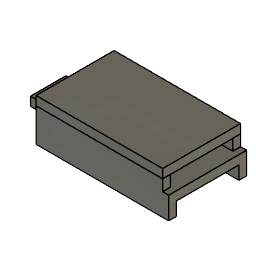
display (Autodesk Fusion 360 design; units mm, degrees)
Autodesk Fusion 360 part; units mm, degrees
note: some values were not read from the file. Chosen so that the rebuilt part matches the saved one: which bodies a step acts on; which face or edge a step refers to. Set by a fixed rule: which sketch regions a step uses.
sketch "スケッチ4" plane through (0, 0, 0) normal (0, 0, 1) x (1, 0, 0)
  line L0 (3, 8.75) -> (3, -8.75)
  line L1 (32.75, -8.75) -> (32.75, 8.75)
  line L2 (5, -8.75) -> (5, 8.75)
  line L3 (3, 8.75) -> (3, -8.75)
  line L4 (-3, -4) -> (-3, 4)
  circle A0 centre (0, 0) radius 1.75
  line L5 (32.75, 8.75) -> (32.75, -8.75)
  line L6 (30.75, 8.75) -> (32.75, 8.75)
  line L7 (32.75, 8.75) -> (3, 8.75)
  line L8 (3, -8.75) -> (32.75, -8.75)
  line L9 (32.75, -8.75) -> (30.75, -8.75)
  line L10 (30.75, -8.75) -> (30.75, 8.75)
  line L11 (-3, 4) -> (3, 4)
  line L12 (3, 4) -> (3, -4)
  line L13 (3, -8.75) -> (5, -8.75)
  line L14 (3, -4) -> (-3, -4)
  line L15 (5, 8.75) -> (3, 8.75)
  line L16 (32.75, 8.75) -> (32.75, -6.75)
  line L17 (3, 8.75) -> (34.75, 8.75)
  line L18 (34.75, 8.75) -> (34.75, 7)
  line L19 (34.75, 7) -> (3, 7)
  line L20 (3, 7) -> (3, 8.75)
  line L21 (30.75, 5) -> (32.75, 5)
  line L22 (32.75, 5) -> (32.75, -7)
  line L23 (32.75, -7) -> (30.75, -7)
  line L24 (30.75, -7) -> (30.75, 5)
  line L25 (3, -8.75) -> (32.75, -8.75)
  line L26 (32.75, -8.75) -> (32.75, -7)
  line L27 (32.75, -7) -> (3, -7)
  line L28 (3, -7) -> (3, -8.75)
  line L29 (34.75, 8.75) -> (31.4, 8.75)
  line L30 (31.4, 8.75) -> (31.4, -8.75)
  line L31 (31.4, -8.75) -> (34.75, -8.75)
  line L32 (34.75, -8.75) -> (34.75, 8.75)
  dimension "d19" = 3.5
  dimension "d20" = 6
  dimension "d21" = 8
  dimension "d22" = 4
  dimension "d23" = 3
  dimension "d24" = 17.5
  dimension "d25" = 8.75
  dimension "d26" = 29.75
  dimension "d33" = 2
  dimension "d34" = 2
  dimension "d35" = 1.75
  dimension "d38" = 2
  dimension "d39" = 1.75
  dimension "d40" = 3.35
  dimension "d41" = 17.5
  constraint coincident A0.centre origin
  constraint horizontal L11
  constraint vertical L12
  constraint horizontal L14
  constraint vertical L4
  constraint horizontal L8
  constraint vertical L1
  constraint horizontal L7
  constraint vertical L3
  constraint collinear L3 L12
  constraint vertical L16
  constraint collinear L1 L16
  constraint horizontal L13
  constraint vertical L2
  constraint horizontal L15
  constraint vertical L0
  constraint horizontal L9
  constraint vertical L10
  constraint horizontal L6
  constraint vertical L5
  constraint collinear L7 L15
  constraint collinear L6 L7
  constraint horizontal L17
  constraint vertical L18
  constraint horizontal L19
  constraint vertical L20
  constraint horizontal L21
  constraint vertical L22
  constraint horizontal L23
  constraint vertical L24
  constraint coincident L16 L22.end
  constraint coincident L10 L21.start
  constraint horizontal L25
  constraint vertical L26
  constraint horizontal L27
  constraint vertical L28
  constraint horizontal L29
  constraint vertical L30
  constraint horizontal L31
  constraint vertical L32
  measures "d19" diameter of A0
  measures "d20" distance of L12.end L4.start
  measures "d21" distance of L4.end L4.start
  measures "d22" distance of A0.centre L14
  measures "d23" distance of A0.centre L4
  measures "d24" distance of L7 L8
  measures "d25" distance of A0.centre L8
  measures "d26" distance of L0.start L1.end
  measures "d33" distance of L2.start L0.end
  measures "d34" distance of L9.end L1.start
  measures "d35" distance of L0.start L19.end
  measures "d38" distance of L19 L21
  measures "d39" distance of L9 L23
  measures "d40" distance of L17.end L29.end
  measures "d41" distance of L17.end L31.end
extrude "押し出し2" add sketch "スケッチ4" along normal blind 5 contours L0 L2 L3 L7 L15 L17 L19 L20 | L0 L2 L3 L12 L19 L27 | L2 L7 L10 L17 L19 | L2 L10 L19 L24 L27 | L6 L7 L10 L17 L19 L30 | L2 L8 L10 L25 L27 | L0 L2 L3 L8 L13 L25 L27 L28 | L10 L19 L21 L30 | L1 L5 L6 L7 L16 L17 L19 L29 L30 | L8 L9 L10 L23 L25 L27 L30 | L10 L21 L23 L24 L27 L30 | L1 L5 L16 L19 L21 L30 | L1 L5 L16 L21 L22 L23 L27 L30 | L1 L5 L8 L9 L23 L25 L26 L27 L30 L31 makes body 1
extrude "押し出し3" add sketch "スケッチ4" along normal blind 9.5 contours L0 L2 L3 L7 L15 L17 L19 L20 | L0 L2 L3 L12 L19 L27 | L2 L7 L10 L17 L19 | L2 L10 L19 L24 L27 | L6 L7 L10 L17 L19 L30 | L2 L8 L10 L25 L27 | L0 L2 L3 L8 L13 L25 L27 L28 | L10 L19 L21 L30 | L8 L9 L10 L23 L25 L27 L30 | L10 L21 L23 L24 L27 L30 bodies 1
extrude "押し出し4" cut sketch "スケッチ4" along normal blind 7.5 contours L0 L2 L3 L12 L19 L27 | L2 L10 L19 L24 L27 | L10 L19 L21 L30 | L10 L21 L23 L24 L27 L30 bodies 1
extrude "押し出し5" add sketch "スケッチ4" along normal blind 5 contours L2 L10 L19 L24 L27 | L10 L19 L21 L30 | L10 L21 L23 L24 L27 L30 bodies 1
extrude "押し出し6" cut sketch "スケッチ4" along normal blind 3 contours L2 L10 L19 L24 L27 | L10 L19 L21 L30 | L10 L21 L23 L24 L27 L30 | L1 L5 L16 L19 L21 L30 | L1 L5 L16 L21 L22 L23 L27 L30 bodies 1
extrude "押し出し7" add sketch "スケッチ4" along normal blind 2 separate body contours L0 L3 L4 L11 L12 L14 makes body 2
extrude "押し出し8" add sketch "スケッチ4" along normal blind 5 contours L0 L2 L3 L12 L19 L27 bodies 1 2
split "分割1" by plane through (0, 0, 7.5) normal (0, 0, -1) bodies 1 makes body 3 at (12.4667, -2.3333, 5)
sketch "スケッチ6" plane through (0, 0, 0) normal (0, 0, -1) x (1, 0, 0)
  circle A0 centre (0, 0) radius 1.75
  line L0 (5, 7) -> (32.75, 7)
  line L1 (32.75, 7) -> (32.75, 8.75)
  line L2 (32.75, 8.75) -> (3, 8.75)
  line L3 (3, 8.75) -> (3, 4)
  line L4 (3, 4) -> (-3, 4)
  line L5 (-3, 4) -> (-3, -4)
  line L6 (-3, -4) -> (3, -4)
  line L7 (3, -4) -> (3, -8.75)
  line L8 (3, -8.75) -> (32.75, -8.75)
  line L9 (32.75, -8.75) -> (32.75, -7)
  line L10 (32.75, -7) -> (5, -7)
  line L11 (5, -7) -> (5, 7)
extrude "押し出し10" add sketch "スケッチ4" along normal blind 4 contours L0 L3 L4 L11 L12 L14 bodies 3
extrude "押し出し11" cut sketch "スケッチ4" along normal blind 2 contours L0 L3 L4 L11 L12 L14 bodies 3
extrude "押し出し1" [suppressed]
equation "d25 = ( 17.5 / 2 ) * 1 mm"
